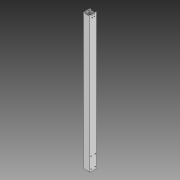
# Autodesk Inventor part: GreyT 2x1 Template
Saved by Autodesk Inventor 2022 (Build 260153000, 153)
## iProperties
Created: 2022-01-01
Part Number: GreyT 2x1 Template
Material: Aluminum 6061
Document SubType Name: Modeling
Density: 2.7 g/cm^3
Appearance: Aluminum - Dark
Autodesk Inventor part; units mm, degrees
ref_plane "YZ Plane" through (0, 0, 0) normal (1, 0, 0) x (0, 1, 0)
ref_plane "XZ Plane" through (0, 0, 0) normal (0, 1, 0) x (-1, 0, 0)
ref_plane "XY Plane" through (0, 0, 0) normal (0, 0, 1) x (1, 0, 0)
sketch "Sketch1" plane through (0, 0, 0) normal (0, 1, 0) x (-1, 0, 0)
  line L0 (-19.05, 19.05) -> (19.05, 19.05)
  line L1 (19.05, 19.05) -> (19.05, -19.05)
  line L2 (19.05, -19.05) -> (-19.05, -19.05)
  line L3 (-19.05, -19.05) -> (-19.05, 19.05)
  line L4 (-19.05, 19.05) -> (19.05, -19.05) construction
  line L5 (19.05, 19.05) -> (-19.05, -19.05) construction
  line L6 (17.4625, -17.4625) -> (17.4625, 17.4625)
  line L7 (17.4625, 17.4625) -> (-17.4625, 17.4625)
  line L8 (-17.4625, 17.4625) -> (-17.4625, -17.4625)
  line L9 (-17.4625, -17.4625) -> (17.4625, -17.4625)
  point P0 (0, 0)
  dimension "d0" = 38.1
  dimension "d1" = 1.5875
  constraints: 20 end point, 4 parallel, 3 perpendicular, 2 midpoint, 1 horizontal, 3 other
  measures "d0" distance of L1.end L2.end
  measures "d1" distance between parallel lines of L1 L6
extrude "Extrusion1" add sketch "Sketch1" along normal mid plane 812.8
sketch "Sketch2" plane through (19.05, -406.4, -19.05) normal (1, 0, 0) x (0, 0, -1)
  circle A0 centre (-25.4, 806.45) radius 2.4892
  circle A1 centre (-25.4, 793.75) radius 2.4892
  circle A2 centre (-12.7, 793.75) radius 2.4892
  circle A3 centre (-12.7, 806.45) radius 2.4892
  line L0 (-38.1, 812.8) -> (0, 812.8) projected
  circle A4 centre (-31.75, 12.7) radius 2.4892
  circle A5 centre (-6.35, 12.7) radius 2.4892
  circle A6 centre (-6.35, 79.375) radius 2.4892
  circle A7 centre (-31.75, 79.375) radius 2.4892
  line L1 (0, 0) -> (-38.1, 0) projected
  line L2 (-38.1, 0) -> (-38.1, 812.8) projected
  point P0 (-19.05, 800.1)
  point P1 (-19.05, 812.8)
  dimension "d4" = 4.9784
  dimension "d7" = 360
  dimension "d9" = 12.7
  dimension "d10" = 6.35
  dimension "d11" = 4.9784
  dimension "d12" = 66.675
  dimension "d13" = 12.7
  dimension "d14" = 25.4
  dimension "d15" = 6.35
  constraints: 8 centre point, 3 equal radius, 3 horizontal alignment, 3 vertical alignment, 1 midpoint, 9 other
  measures "d4" diameter of A0
  measures "d9" distance of A3.centre A0.centre
  measures "d10" distance from line of L0 A0.centre
  measures "d11" diameter of A4
  measures "d12" distance of A4.centre A7.centre
  measures "d13" distance from line of L1 A4.centre
  measures "d14" distance of A5.centre A4.centre
  measures "d15" distance from line of L2 A4.centre
extrude "Extrusion2" cut sketch "Sketch2" against normal through all
sketch "Sketch3" plane through (-19.05, 406.4, 19.05) normal (0, 0, 1) x (1, 0, 0)
  line L0 (0, 0) -> (38.1, 0) projected
  line L1 (7.9375, 0) -> (7.9375, -6.35)
  line L2 (7.9375, -6.35) -> (30.1625, -6.35)
  line L3 (30.1625, -6.35) -> (30.1625, 0)
  point P0 (19.05, -6.35)
  point P1 (19.05, 0)
  dimension "d18" = 22.225
  dimension "d19" = 6.35
  constraints: 6 end point, 2 midpoint, 2 perpendicular, 2 point on line, 1 vertical, 1 vertical alignment
  measures "d18" distance of L1.end L2.end
  measures "d19" distance of L1.start L1.end
extrude "Extrusion3" cut sketch "Sketch3" against normal through all
fillet "Fillet1" radius 2.54 8 edges at (-11.1125, 406.4, 18.2562) (-11.1125, 400.05, 18.2562) (11.1125, 400.05, 18.2562) (11.1125, 406.4, 18.2562) (-11.1125, 406.4, -18.2562) (-11.1125, 400.05, -18.2562) (11.1125, 406.4, -18.2562) (11.1125, 400.05, -18.2562)
body "Solid1"
